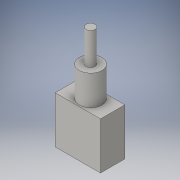
# Autodesk Inventor part: Aidan Sherry Switch
Saved by Autodesk Inventor 2016 (Build 200138000, 138)
## iProperties
Created: 2016-10-05
Part Number: Aidan Sherry Switch
Material: Generic
Document SubType Name: Modeling
Designer: sherra
Density: 1 g/cm^3
Appearance: Default
Author: sherra
Autodesk Inventor part; units mm, degrees
ref_plane "YZ Plane" through (0, 0, 0) normal (1, 0, 0) x (0, 1, 0)
ref_plane "XZ Plane" through (0, 0, 0) normal (0, 1, 0) x (-1, 0, 0)
ref_plane "XY Plane" through (0, 0, 0) normal (0, 0, 1) x (1, 0, 0)
sketch "Sketch1" plane through (0, 0, 0) normal (0, 0, 1) x (1, 0, 0)
  line L0 (-5.9795, 4.5091) -> (6.9237, 4.5091)
  line L1 (6.9237, 4.5091) -> (6.9237, -8.8513)
  line L2 (6.9237, -8.8513) -> (-5.9795, -8.8513)
  line L3 (-5.9795, -8.8513) -> (-5.9795, 4.5091)
  point P0 (0, 0)
  dimension "d0" = 12.9032
  dimension "d1" = 13.3604
  constraints: 8 end point, 2 parallel, 1 horizontal, 1 perpendicular
  measures "d0" distance between parallel lines of L1 L3
  measures "d1" distance between parallel lines of L2 L0
extrude "Extrusion1" add sketch "Sketch1" along normal blind 6.9342
sketch "Sketch2" plane through (-5.9795, 4.5091, 0) normal (0, 1, 0) x (1, 0, 0)
  circle A0 centre (6.4761, -3.3308) radius 3.2234
  point P0 (5.9795, 0)
  dimension "d4" = 6.4469
  constraints: 1 centre point
  measures "d4" diameter of A0
extrude "Extrusion2" add sketch "Sketch2" along normal blind 8.5344
sketch "Sketch3" plane through (0.4966, 13.0435, 3.3308) normal (0, 1, 0) x (1, 0, 0)
  circle A0 centre (0, 0) radius 1.27
  point P0 (-0.4966, 3.3308)
  dimension "d7" = 2.54
  constraints: 1 centre point
  measures "d7" diameter of A0
extrude "Extrusion3" add sketch "Sketch3" along normal blind 9.144
sketch "Sketch4" plane through (-5.9795, -8.8513, 0) normal (-1, 0, 0) x (0, 0, 1)
  point P0 (0, 8.8513)
body "Solid1"
